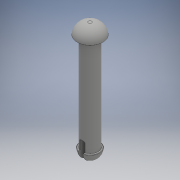
# Autodesk Inventor part: N4049_pìno_tampa_superior
Saved by Autodesk Inventor 2018 (Build 220112000, 112)
## iProperties
Created: 2021-03-23
Part Number: N4049_pìno_tampa_superior
Material: Genérico
Document SubType Name: Modeling
Designer: nilton
Density: 1 g/cm^3
Appearance: Cinza claro
Author: nilton
Autodesk Inventor part; units mm, degrees
ref_plane "YZ Plane" through (0, 0, 0) normal (1, 0, 0) x (0, 1, 0)
ref_plane "XZ Plane" through (0, 0, 0) normal (0, 1, 0) x (-1, 0, 0)
ref_plane "XY Plane" through (0, 0, 0) normal (0, 0, 1) x (1, 0, 0)
sketch "Esboço1" plane through (0, 0, 0) normal (0, 0, 1) x (1, 0, 0)
  circle A0 centre (0, 0) radius 2.5
  dimension "d0" = 5
  constraints: 1 centre point, 1 coincident
  measures "d0" diameter of A0
extrude "Extrusão1" add sketch "Esboço1" along normal mid plane 30
sketch "Esboço2" plane through (0, 0, 15) normal (0, 0, 1) x (1, 0, 0)
  circle A0 centre (0, 0) radius 2.5 projected
  circle A1 centre (0, 0) radius 4
  dimension "d3" = 8
  constraints: 1 centre point, 1 coincident
  measures "d3" diameter of A1
extrude "Extrusão2" add sketch "Esboço2" along normal blind 3.5 contours A0 | A1
fillet "Arredondamento1" radius 3.5 1 edges at (-4, 0, 18.5)
sketch "Esboço3" plane through (0, 0, -15) normal (0, 0, -1) x (-1, 0, 0)
  circle A0 centre (0, 0) radius 3
  dimension "d7" = 6
  constraints: 1 centre point, 1 coincident
  measures "d7" diameter of A0
extrude "Extrusão3" add sketch "Esboço3" along normal blind 3
fillet "Arredondamento2" radius 3 1 edges at (3, 0, -18)
sketch "Esboço4" plane through (0, 0, 0) normal (1, 0, 0) x (0, 1, 0)
  line L0 (-2.5, -15) -> (-2.5, 15) projected
  line L1 (2.5, -15) -> (2.5, 15) projected
  arc A0 (-3, -15) -> (3, -15) centre (0, -15) ccw projected
  line L2 (3, -15) -> (-3, -15) projected
  line L3 (-3, -18) -> (3, -18)
  line L4 (3, -18) -> (3, -12)
  line L5 (3, -12) -> (-3, -12)
  line L6 (-3, -12) -> (-3, -18)
  point P0 (0, 0)
  point P1 (0, -18)
  dimension "d11" = 6
  constraints: 8 end point, 2 midpoint, 2 parallel, 1 horizontal, 1 perpendicular, 1 point on circle
  measures "d11" distance from line of L5 point (0, -18)
extrude "Extrusão4" cut sketch "Esboço4" along normal mid plane 1.5 contours L2 L6 L5 L0 | L0 L5 L1 L2 | L2 A0 | L1 L5 L4 L2 | L4 L3 A0
fillet "Arredondamento3" radius 0.5 2 edges at (-0.75, 0, -12) (0.75, 0, -12)
fillet "Arredondamento4" radius 0.1 15 edges at (0.6098, -2.4245, -12.1528) (0.6098, 2.4245, -12.1528) (0, -2.5, -12) (0, 2.5, -12) (-0.6098, -2.4245, -12.1528) (-0.6098, 2.4245, -12.1528) (-0.75, 2.3848, -13.75) (-0.75, -2.3848, -13.75) (0.75, -2.3848, -13.75) (0.75, 2.3848, -13.75) (3, 0, -15.0001) (-3, 0, -15) (-3, 0, -15.0001) (-4, 0, 15) (-4, 0, 15.0001)
